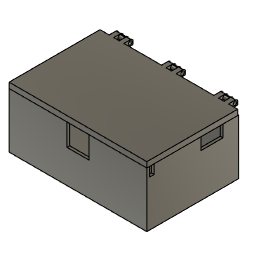
垃圾桶 (Autodesk Fusion 360 design; units mm, degrees)
part number: 2025-05-22-16-17-18-557
part number: 2025-05-22-16-22-29-494
part number: 2025-05-22-17-19-36-392
Autodesk Fusion 360 part; units mm, degrees
sketch "草图1" plane through (0, 0, 0) normal (0, 0, 1) x (1, 0, 0)
  line L0 (0, 0) -> (150, 0)
  line L1 (150, 0) -> (150, 100)
  line L2 (150, 100) -> (0, 100)
  line L3 (0, 100) -> (0, 0)
  dimension "d1" = 150
  dimension "d2" = 100
  constraint horizontal L0
  constraint vertical L1
  constraint horizontal L2
  constraint vertical L3
  constraint coincident L0.start L3.end
  measures "d1" distance of L0.start L0.end
  measures "d2" distance of L0.start L2.end
extrude "拉伸1" add sketch "草图1" along normal blind 3 makes body 1 in component "Component'"
sketch "草图2" plane through (0, 0, 3) normal (0, 0, 1) x (-1, 0, 0)
  line L0 (0, -100) -> (0, 0)
  line L1 (0, 0) -> (-150, 0)
  line L2 (-150, 0) -> (-150, -100)
  line L3 (-150, -100) -> (0, -100)
  line L4 (-3, -3) -> (-147, -3)
  line L5 (-147, -3) -> (-147, -97)
  line L6 (-147, -97) -> (-3, -97)
  line L7 (-3, -97) -> (-3, -3)
  dimension "d6" = -3
extrude "拉伸2" add sketch "草图2" along normal blind 97 bodies 1 in component "Component'"
sketch "草图3" plane through (0, 0, 0) normal (0, -1, 0) x (1, 0, 0)
  line L0 (0, 0) -> (150, 0)
  line L1 (150, 0) -> (150, 100)
  line L2 (150, 100) -> (0, 100)
  line L3 (0, 100) -> (0, 0)
  line L4 (63, 100) -> (87, 100)
  line L5 (87, 100) -> (87, 76)
  line L6 (87, 76) -> (63, 76)
  line L7 (63, 76) -> (63, 100)
  dimension "d9" = 24
  dimension "d10" = 24
  constraint horizontal L4
  constraint vertical L5
  constraint horizontal L6
  constraint vertical L7
  constraint midpoint L2 L4
  measures "d9" distance of L4.start L4.end
  measures "d10" distance of L4.start L6.end
extrude "拉伸3" cut sketch "草图3" against normal blind 25 contours L2 L4 L5 L6 L7 bodies 1 in component "Component'"
sketch "草图4" plane through (0, 0, 0) normal (-1, 0, 0) x (0, -1, 0)
  line L0 (-100, 0) -> (0, 0)
  line L1 (0, 0) -> (0, 100)
  line L2 (0, 100) -> (-100, 100)
  line L3 (-100, 100) -> (-100, 0)
  line L4 (-71, 100) -> (-54.5, 100)
  line L5 (-54.5, 100) -> (-54.5, 83.5)
  line L6 (-54.5, 83.5) -> (-71, 83.5)
  line L7 (-71, 83.5) -> (-71, 100)
  line L8 (-45.5, 100) -> (-29, 100)
  line L9 (-29, 100) -> (-29, 83.5)
  line L10 (-29, 83.5) -> (-45.5, 83.5)
  line L11 (-45.5, 83.5) -> (-45.5, 100)
  line L12 (-54.5, 100) -> (-45.5, 100) construction
  line L13 (-54.5, 100) -> (-45.5, 100)
  line L14 (-45.5, 100) -> (-45.5, 97.5)
  line L15 (-45.5, 97.5) -> (-54.5, 97.5)
  line L16 (-54.5, 97.5) -> (-54.5, 100)
  dimension "d13" = 16.5
  dimension "d14" = 16.5
  dimension "d15" = 16.5
  dimension "d16" = 16.5
  dimension "d17" = 9
  dimension "d18" = 14
  constraint horizontal L4
  constraint vertical L5
  constraint horizontal L6
  constraint vertical L7
  constraint horizontal L8
  constraint vertical L9
  constraint horizontal L10
  constraint vertical L11
  constraint collinear L4 L8
  constraint midpoint L2 L12
  constraint horizontal L13
  constraint vertical L14
  constraint horizontal L15
  constraint vertical L16
  constraint coincident L11 L14.end
  measures "d13" distance of L4.start L4.end
  measures "d14" distance of L4.start L6.end
  measures "d15" distance of L8.start L8.end
  measures "d16" distance of L8.start L10.end
  measures "d17" distance of L5 L11
  measures "d18" distance of L6 L15
extrude "拉伸4" cut sketch "草图4" against normal blind 10 contours L2 L4 L5 L6 L7 L16 | L2 L8 L9 L10 L11 L14 | L2 L5 L11 L13 L14 L15 L16 bodies 1 in component "Component'"
sketch "草图5" plane through (150, 0, 0) normal (1, 0, 0) x (0, 1, 0)
  line L0 (0, 0) -> (100, 0)
  line L1 (100, 0) -> (100, 100)
  line L2 (100, 100) -> (0, 100)
  line L3 (0, 100) -> (0, 0)
  line L4 (59, 100) -> (83, 100)
  line L5 (83, 100) -> (83, 87)
  line L6 (83, 87) -> (59, 87)
  line L7 (59, 87) -> (59, 100)
  dimension "d21" = 24
  dimension "d22" = 13
  dimension "d23" = 17
  constraint horizontal L4
  constraint vertical L5
  constraint horizontal L6
  constraint vertical L7
  constraint coincident L2 L4.start
  measures "d21" distance of L4.start L4.end
  measures "d22" distance of L4.start L6.end
  measures "d23" distance of L1 L5
extrude "拉伸5" cut sketch "草图5" against normal blind 20 contours L2 L4 L5 L6 L7 bodies 1 in component "Component'"
sketch "草图6" plane through (147, 0, 0) normal (-1, 0, 0) x (0, -1, 0)
  line L0 (-59, 100) -> (-59, 87)
  line L1 (-59, 87) -> (-83, 87)
  line L2 (-83, 87) -> (-83, 100)
  line L3 (-83, 100) -> (-97, 100)
  line L4 (-97, 100) -> (-97, 3)
  line L5 (-97, 3) -> (-3, 3)
  line L6 (-3, 3) -> (-3, 100)
  line L7 (-3, 100) -> (-59, 100)
  line L8 (-8, 100) -> (-3, 100)
  line L9 (-3, 100) -> (-3, 90)
  line L10 (-3, 90) -> (-8, 90)
  line L11 (-8, 90) -> (-8, 100)
  dimension "d26" = 5
  dimension "d27" = 10
  constraint horizontal L8
  constraint vertical L9
  constraint horizontal L10
  constraint vertical L11
  constraint coincident L7 L8.start
  constraint collinear L6 L9
  measures "d26" distance of L8.start L6.end
  measures "d27" distance of L8.start L10.end
extrude "拉伸6" cut sketch "草图6" against normal blind 10 contours L6 L7 L8 L9 L10 L11 bodies 1 in component "Component'"
ref_plane "工作平面1" through (75, 50, 50) normal (1, 0, 0) x (0, 1, 0)
sketch "草图7" plane through (75, 0, 0) normal (1, 0, 0) x (0, 1, 0)
  line L0 (100, 100) -> (103, 100)
  line L1 (103, 100) -> (103, 103.5)
  line L2 (105.5, 106) -> (106.5, 106)
  line L3 (109, 103.5) -> (109, 100)
  line L4 (108.7423, 99.3777) -> (100, 90.6355)
  circle A0 centre (106, 103) radius 2
  line L5 (100, 0) -> (100, 100)
  arc A1 (105.5, 106) -> (103, 103.5) centre (105.5, 103.5) ccw
  arc A2 (109, 103.5) -> (106.5, 106) centre (106.5, 103.5) ccw
  arc A3 (108.7423, 99.3777) -> (109, 100) centre (108.12, 100) ccw
  point P0 (100, 100)
  dimension "d30" = 3
  dimension "d31" = 4
  dimension "d32" = 3
  dimension "d33" = 3
  dimension "d34" = 3
  dimension "d35" = 3
  dimension "d36" = 135
  dimension "d37" = 2.5
  dimension "d38" = 2.5
  dimension "d39" = 0.88
  constraint horizontal L0
  constraint perpendicular L0 L1
  constraint perpendicular L1 L2
  constraint perpendicular L2 L3
  constraint coincident P0 L0.start
  constraint coincident L4.end L5
  constraint tangent L2 A1
  constraint tangent L1 A1
  constraint tangent L2 A2
  constraint tangent L3 A2
  constraint tangent L3 A3
  constraint tangent L4 A3
  constraint equal L1 L3
  measures "d30" distance of P0 L0.end
  measures "d31" diameter of A0
  measures "d32" distance of L1 A0.centre
  measures "d33" distance of L3 A0.centre
  measures "d34" distance of L2 A0.centre
  measures "d35" vertical distance of L0.end A0.centre
  measures "d36" angle of L3 L4
  measures "d37" radius of A1
  measures "d38" radius of A2
  measures "d39" radius of A3
extrude "拉伸7" add sketch "草图7" along normal mid plane 5 bodies 1 in component "Component'"
ref_plane "工作平面2" through (18, 50, 51.5) normal (1, 0, 0) x (0, 1, 0)
sketch "草图8" plane through (18, 0, 0) normal (1, 0, 0) x (0, 1, 0)
  arc A0 (108.7423, 99.3777) -> (109, 100) centre (108.12, 100) ccw
  arc A1 (105.5, 106) -> (103, 103.5) centre (105.5, 103.5) ccw
  line L0 (105.5, 106) -> (106.5, 106)
  line L1 (100, 100) -> (103, 100)
  arc A2 (109, 103.5) -> (106.5, 106) centre (106.5, 103.5) ccw
  circle A3 centre (106, 103) radius 2
  line L2 (109, 103.5) -> (109, 100)
  line L3 (108.7423, 99.3777) -> (100, 90.6355)
  line L4 (103, 100) -> (103, 103.5)
  line L5 (100, 0) -> (100, 100)
  point P0 (100, 100)
  point P1 (100, 100)
  point P2 (100, 100)
  dimension "d43" = 3
  dimension "d44" = 4
  dimension "d45" = 3
  dimension "d46" = 3
  dimension "d47" = 3
  dimension "d48" = 3
  dimension "d49" = 135
  dimension "d50" = 2.5
  dimension "d51" = 2.5
  dimension "d52" = 0.88
  constraint horizontal L1
  constraint perpendicular L1 L4
  constraint perpendicular L0 L4
  constraint perpendicular L0 L2
  constraint coincident P2 P1
  constraint tangent A1 L0
  constraint tangent A1 L4
  constraint tangent L0 A2
  constraint tangent A2 L2
  constraint tangent A0 L2
  constraint tangent A0 L3
  constraint equal L2 L4
  constraint coincident L3.end L5
  measures "d43" distance of L1.end P2
  measures "d44" diameter of A3
  measures "d45" distance of A3.centre L4
  measures "d46" distance of A3.centre L2
  measures "d47" distance of A3.centre L0
  measures "d48" vertical distance of L1.end A3.centre
  measures "d49" angle of L2 L3
  measures "d50" radius of A1
  measures "d51" radius of A2
  measures "d52" radius of A0
ref_plane "工作平面3" through (132, 50, 51.5) normal (-1, 0, 0) x (0, -1, 0)
sketch "草图9" plane through (132, 0, 0) normal (-1, 0, 0) x (0, -1, 0)
extrude "拉伸8" add sketch "草图8" along normal mid plane 5 bodies 1 in component "Component'"
ref_plane "工作平面4" through (132, 50, 51.5) normal (-1, 0, 0) x (0, -1, 0)
sketch "草图10" plane through (132, 0, 0) normal (-1, 0, 0) x (0, -1, 0)
  line L0 (-100, 100) -> (-103, 100)
  line L1 (-105.5, 106) -> (-106.5, 106)
  arc A0 (-106.5, 106) -> (-109, 103.5) centre (-106.5, 103.5) ccw
  line L2 (-103, 100) -> (-103, 103.5)
  arc A1 (-103, 103.5) -> (-105.5, 106) centre (-105.5, 103.5) ccw
  circle A2 centre (-106, 103) radius 2
  line L3 (-109, 103.5) -> (-109, 100)
  arc A3 (-109, 100) -> (-108.7657, 99.4343) centre (-108.2, 100) ccw
  line L4 (-108.7657, 99.4343) -> (-100, 90.6686)
  line L5 (-100, 0) -> (-100, 100)
  point P0 (-105.9337, 94.2405)
  point P1 (-105.9337, 94.2405)
  point P2 (-100, 100)
  dimension "d67" = 3.5
  dimension "d68" = 3
  dimension "d69" = 3
  dimension "d70" = 3
  dimension "d71" = 3
  dimension "d72" = 3
  dimension "d73" = 1
  dimension "d74" = 4
  dimension "d75" = 0.8
  dimension "d76" = 135
  constraint equal L2 L3
  constraint horizontal L1
  constraint vertical L2
  constraint tangent L1 A1
  constraint tangent L1 A0
  constraint tangent L2 A1
  constraint tangent A0 L3
  constraint tangent L3 A3
  constraint tangent A3 L4
  constraint perpendicular L0 L2
  constraint coincident P2 L0.start
  constraint coincident L4.end L5
  constraint vertical L3
  measures "d67" distance of L0.end L2.end
  measures "d68" distance of P2 L0.end
  measures "d69" distance of A2.centre L2
  measures "d70" distance of A2.centre L1
  measures "d71" distance of A2.centre L3
  measures "d72" vertical distance of L0.end A2.centre
  measures "d73" distance of L1.start L1.end
  measures "d74" diameter of A2
  measures "d75" radius of A3
  measures "d76" angle of L3 L4
extrude "拉伸9" add sketch "草图10" along normal mid plane 5 bodies 1 in component "Component'"
sketch "草图11" plane through (0, 0, 100) normal (0, 0, 1) x (-1, 0, 0)
  line L0 (-3, -29) -> (0, -29)
  line L1 (0, -29) -> (0, 0)
  line L2 (0, 0) -> (-63, 0)
  line L3 (-63, 0) -> (-63, -3)
  line L4 (-63, -3) -> (-3, -3)
  line L5 (-3, -3) -> (-3, -29)
  line L6 (0, -109) -> (-150, -109)
  line L7 (-150, -109) -> (-150, 0)
  line L8 (-150, 0) -> (0, 0)
  line L9 (0, 0) -> (0, -109)
  dimension "d79" = 150
  dimension "d80" = 109
  constraint horizontal L6
  constraint vertical L7
  constraint horizontal L8
  constraint vertical L9
  constraint coincident L1.end L2.start
  measures "d79" distance of L6.start L6.end
  measures "d80" distance of L6.start L1.end
extrude "拉伸1'" add sketch "草图11" along normal blind 6 separate body makes body 2 in component "Component''"
sketch "草图12" plane through (0, 0, 106) normal (0, 0, 1) x (-1, 0, 0)
  line L0 (0, 0) -> (-150, 0)
  line L1 (-150, 0) -> (-150, -109)
  line L2 (-150, -109) -> (0, -109)
  line L3 (0, -109) -> (0, 0)
  line L4 (-135, -99) -> (-129, -99)
  line L5 (-129, -99) -> (-129, -109)
  line L6 (-129, -109) -> (-135, -109)
  line L7 (-135, -109) -> (-135, -99)
  line L8 (-78, -99) -> (-72, -99)
  line L9 (-72, -99) -> (-72, -109)
  line L10 (-72, -109) -> (-78, -109)
  line L11 (-78, -109) -> (-78, -99)
  line L12 (-21, -99) -> (-15, -99)
  line L13 (-15, -99) -> (-15, -109)
  line L14 (-15, -109) -> (-21, -109)
  line L15 (-21, -109) -> (-21, -99)
  dimension "d83" = 6
  dimension "d84" = 10
  dimension "d85" = 15
  dimension "d86" = 6
  dimension "d87" = 10
  dimension "d88" = 6
  dimension "d89" = 10
  dimension "d90" = 72
  dimension "d91" = 15
  constraint horizontal L4
  constraint vertical L5
  constraint horizontal L6
  constraint vertical L7
  constraint collinear L2 L6
  constraint horizontal L8
  constraint vertical L9
  constraint horizontal L10
  constraint vertical L11
  constraint horizontal L12
  constraint vertical L13
  constraint horizontal L14
  constraint vertical L15
  constraint collinear L2 L10
  constraint collinear L2 L14
  measures "d83" distance of L4.start L4.end
  measures "d84" distance of L4.start L6.end
  measures "d85" distance of L1 L7
  measures "d86" distance of L8.start L8.end
  measures "d87" distance of L8.start L10.end
  measures "d88" distance of L12.start L12.end
  measures "d89" distance of L12.start L14.end
  measures "d90" distance of L1 L11
  measures "d91" distance of L3 L13
extrude "拉伸2'" cut sketch "草图12" against normal blind 10 contours L2 L12 L13 L14 L15 | L2 L4 L5 L6 L7 | L2 L8 L9 L10 L11 bodies 2 in component "Component''"
sketch "草图13" plane through (150, 0, 0) normal (1, 0, 0) x (0, 1, 0)
  line L0 (0, 100) -> (109, 100)
  line L1 (109, 100) -> (109, 106)
  line L2 (109, 106) -> (0, 106)
  line L3 (0, 106) -> (0, 100)
  circle A0 centre (106, 103) radius 2
  dimension "d94" = 4
  dimension "d95" = 3
  dimension "d96" = 3
  measures "d94" diameter of A0
  measures "d95" distance of L1 A0.centre
  measures "d96" distance of L2 A0.centre
extrude "拉伸3'" cut sketch "草图13" against normal blind 170 contours A0 bodies 2 in component "Component''"
fillet "圆角1" radius 2.5 4 edges at (142.5, 109, 106) (103.5, 109, 106) (46.5, 109, 106) (7.5, 109, 106) on bodies 2 in component "Component''"
extrude "拉伸10" add 1 faces at (51, 65.6667, 3) along direction (0, 0, 1) blind 40 on bodies 1 bodies 1 in component "Component'"
extrude "拉伸11" cut 1 faces at (50, 66.6667, 0) along direction (0, 0, 1) blind 40 on bodies 1 bodies 1 in component "Component'"
sketch "草图14" plane through (0, 0, 13.3714) normal (0, 0, 1) x (-1, 0, 0)
  line L0 (10.9987, -232.8503) -> (25.9987, -232.8503)
  line L1 (25.9987, -232.8503) -> (25.9987, -126.3503)
  line L2 (25.9987, -126.3503) -> (-124.0013, -126.3503)
  line L3 (-124.0013, -126.3503) -> (-124.0013, -232.8503)
  line L4 (-124.0013, -232.8503) -> (-109.0013, -232.8503)
  line L5 (-109.0013, -232.8503) -> (-109.0013, -225.3503)
  line L6 (-109.0013, -225.3503) -> (-103.0013, -225.3503)
  line L7 (-103.0013, -225.3503) -> (-103.0013, -232.8503)
  line L8 (-103.0013, -232.8503) -> (-52.0013, -232.8503)
  line L9 (-52.0013, -232.8503) -> (-52.0013, -225.3503)
  line L10 (-52.0013, -225.3503) -> (-46.0013, -225.3503)
  line L11 (-46.0013, -225.3503) -> (-46.0013, -232.8503)
  line L12 (-46.0013, -232.8503) -> (4.9987, -232.8503)
  line L13 (4.9987, -232.8503) -> (4.9987, -225.3503)
  line L14 (4.9987, -225.3503) -> (10.9987, -225.3503)
  line L15 (10.9987, -225.3503) -> (10.9987, -232.8503)
  line L16 (-114.0013, -225.3503) -> (-127.4522, -225.3503)
  line L17 (-127.4522, -225.3503) -> (-127.4522, -236.557)
  line L18 (-127.4522, -236.557) -> (-114.0013, -236.557)
  line L19 (-114.0013, -236.557) -> (-114.0013, -225.3503)
  line L20 (-98.0013, -225.3503) -> (-57.0013, -225.3503)
  line L21 (-57.0013, -225.3503) -> (-57.0013, -239)
  line L22 (-57.0013, -239) -> (-98.0013, -239)
  line L23 (-98.0013, -239) -> (-98.0013, -225.3503)
  line L24 (-41.0013, -225.3503) -> (-0.0013, -225.3503)
  line L25 (-0.0013, -225.3503) -> (-0.0013, -240)
  line L26 (-0.0013, -240) -> (-41.0013, -240)
  line L27 (-41.0013, -240) -> (-41.0013, -225.3503)
  line L28 (15.9987, -225.3503) -> (29.1278, -225.3503)
  line L29 (29.1278, -225.3503) -> (29.1278, -239)
  line L30 (29.1278, -239) -> (15.9987, -239)
  line L31 (15.9987, -239) -> (15.9987, -225.3503)
  dimension "d105" = 5
  dimension "d106" = 5
  dimension "d107" = 5
  dimension "d108" = 5
  dimension "d109" = 5
  dimension "d110" = 5
  constraint horizontal L16
  constraint vertical L17
  constraint horizontal L18
  constraint vertical L19
  constraint collinear L6 L16
  constraint horizontal L20
  constraint vertical L21
  constraint horizontal L22
  constraint vertical L23
  constraint horizontal L24
  constraint vertical L25
  constraint horizontal L26
  constraint vertical L27
  constraint horizontal L28
  constraint vertical L29
  constraint horizontal L30
  constraint vertical L31
  measures "d105" distance of L5 L19
  measures "d106" distance of L7 L23
  measures "d107" distance of L9 L21
  measures "d108" distance of L11 L27
  measures "d109" distance of L13 L25
  measures "d110" distance of L15 L31
extrude "拉伸4'" cut sketch "草图14" against normal blind 25 contours L0 L1 L28 L31 | L0 L1 L28 L29 L30 L31 | L12 L25 L26 L27 | L12 L24 L25 L27 | L3 L4 L16 L19 | L3 L4 L16 L17 L18 L19 | L8 L21 L22 L23 | L8 L20 L21 L23 sketch seen with x (1, 0, 0) y (0, 1, 0) z (0, 0, 1) at (25.9987, -126.3503, 92.6286) bodies 2 in component "Component''"
component "Component'" placed x (1, 0, 0) y (0, 1, 0) z (0, 0, 1) at (0, 0, 0)
component "Component''" placed x (1, 0, 0) y (0, 1, 0) z (0, 0, 1) at (0, 0, 0)
equation "d7 = 100 mm - 3 mm"
